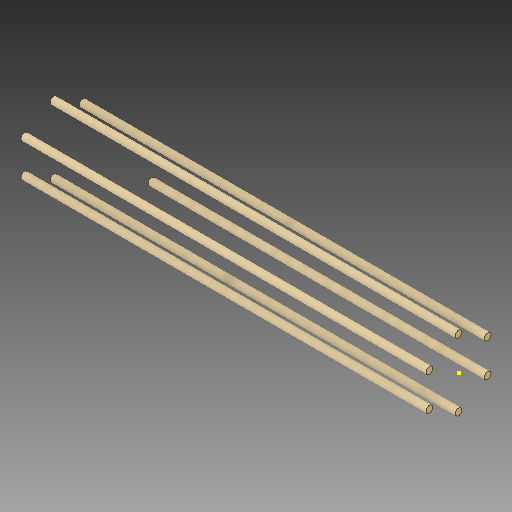
# Autodesk Inventor part: Ceramic Support
Saved by Autodesk Inventor 2017.3 (Build 213256000, 256)
## iProperties
Created: 2017-02-02
Part Number: Ceramic Support
Material: Generic
Document SubType Name: Modeling
Designer: Mac
Density: 1 g/cm^3
Appearance: Wheat
Author: Mac
Autodesk Inventor part; units mm, degrees
ref_plane "YZ Plane" through (0, 0, 0) normal (1, 0, 0) x (0, 1, 0)
ref_plane "XZ Plane" through (0, 0, 0) normal (0, 1, 0) x (-1, 0, 0)
ref_plane "XY Plane" through (0, 0, 0) normal (0, 0, 1) x (1, 0, 0)
sketch "Sketch1" plane through (0, 0, 0) normal (1, 0, 0) x (0, 1, 0)
  circle A0 centre (0, 0) radius 9.5
  dimension "d0" = 19
  constraints: 1 centre point, 1 coincident
  measures "d0" diameter of A0
extrude "Extrusion1" add sketch "Sketch1" along normal blind 1
sketch "Sketch2" plane through (1, 0, 0) normal (1, 0, 0) x (0, 0, -1)
  circle A0 centre (0, 7.81) radius 0.8
  circle A1 centre (0, -7.81) radius 0.8
  circle A2 centre (6.7637, 3.905) radius 0.8
  circle A3 centre (6.7637, -3.905) radius 0.8
  circle A4 centre (-6.7637, -3.905) radius 0.8
  circle A5 centre (-6.7637, 3.905) radius 0.8
  point P0 (0, 0)
  dimension "d4" = 1.6
  dimension "d5" = 1.6
  dimension "d6" = 1.6
  dimension "d7" = 1.6
  dimension "d8" = 1.6
  dimension "d9" = 1.6
  constraints: 6 centre point
  measures "d4" diameter of A0
  measures "d5" diameter of A1
  measures "d6" diameter of A2
  measures "d7" diameter of A3
  measures "d8" diameter of A4
  measures "d9" diameter of A5
extrude "Extrusion2" add sketch "Sketch2" along normal blind 99
sketch "Sketch3" plane through (100, -3.905, 6.7637) normal (1, 0, 0) x (0, 0, -1)
  point P0 (6.7637, 3.905)
sketch "Sketch4" plane through (0, 0, 0) normal (-1, 0, 0) x (0, 0, 1)
  circle A0 centre (0, 0) radius 10
  constraints: 1 centre point, 1 coincident
extrude "Extrusion3" cut sketch "Sketch4" against normal blind 6
sketch "Sketch5" plane through (6, -3.905, -6.7637) normal (-1, 0, 0) x (0, 0, 1)
  circle A0 centre (0, 0) radius 0.8 projected
  circle A1 centre (0, 0) radius 2.3412
  point P0 (6.7637, 3.905)
  constraints: 1 centre point, 1 coincident
extrude "Extrusion4" cut sketch "Sketch5" against normal blind 16 contours A0
body "Solid1"
